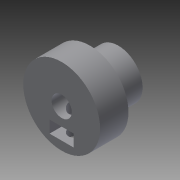
# Autodesk Inventor part: штука от моторчика2015
Saved by Autodesk Inventor 2015 (Build 190159000, 159)
## iProperties
Created: 2016-04-10
Part Number: штука от моторчика2015
Material: Generic
Document SubType Name: Modeling
Designer: 1
Density: 1 g/cm^3
Appearance: Default
Author: 1
Autodesk Inventor part; units mm, degrees
ref_plane "YZ Plane" through (0, 0, 0) normal (1, 0, 0) x (0, 1, 0)
ref_plane "XZ Plane" through (0, 0, 0) normal (0, 1, 0) x (-1, 0, 0)
ref_plane "XY Plane" through (0, 0, 0) normal (0, 0, 1) x (1, 0, 0)
sketch "Sketch1" plane through (0, 0, 0) normal (0, 1, 0) x (-1, 0, 0)
  circle A0 centre (0, 0) radius 6
  dimension "d0" = 12
  constraints: 1 centre point, 1 coincident
  measures "d0" diameter of A0
extrude "Extrusion1" add sketch "Sketch1" along normal blind 4 and the other way blind 3
sketch "Sketch2" plane through (0, -3, 0) normal (0, -1, 0) x (1, 0, 0)
  circle A0 centre (0, 0) radius 9.5
  dimension "d3" = 19
  constraints: 1 centre point, 1 coincident
  measures "d3" diameter of A0
extrude "Extrusion2" add sketch "Sketch2" along normal blind 7
sketch "Sketch7" plane through (0, 0, 0) normal (0, 0, 1) x (1, 0, 0)
  point P0 (0, 0)
sketch "Sketch9" plane through (0, 0, 0) normal (0, 0, 1) x (1, 0, 0)
  circle A0 centre (0, -6.5) radius 1.75
  line L0 (-9.5, -10) -> (9.5, -10) projected
  line L1 (0, -10) -> (0, -3)
  line L2 (0, -10) -> (0, -3)
  line L3 (-6, -3) -> (6, -3) projected
  point P0 (0, 0)
  dimension "d22" = 3.5
  constraints: 4 end point, 4 midpoint, 1 centre point, 1 coincident, 1 perpendicular
  measures "d22" diameter of A0
extrude "Extrusion8" cut sketch "Sketch9" against normal up to next
sketch "Sketch10" plane through (0, 4, 0) normal (0, 1, 0) x (1, 0, 0)
  circle A0 centre (0, 0) radius 2.5
  dimension "d26" = 5
  constraints: 1 centre point, 1 coincident
  measures "d26" diameter of A0
extrude "Extrusion9" cut sketch "Sketch10" against normal through all
sketch "Sketch11" plane through (0, -10, 0) normal (0, -1, 0) x (1, 0, 0)
  line L0 (3, -7.3359) -> (-3, -7.3359)
  line L1 (-3, -7.3359) -> (-3, -4.3359)
  line L2 (-3, -4.3359) -> (3, -4.3359)
  line L3 (3, -4.3359) -> (3, -7.3359)
  circle A0 centre (0, 0) radius 9.5 projected
  circle A1 centre (0, 0) radius 2.5 projected
  line L4 (0, -2.5) -> (0, -9.5)
  line L5 (4.4339, -2.3359) -> (-4.4946, -2.3359)
  line L6 (-4.4946, -2.3359) -> (-4.4946, -9.3359)
  line L7 (-4.4946, -9.3359) -> (4.4339, -9.3359)
  line L8 (4.4339, -9.3359) -> (4.4339, -2.3359)
  line L9 (-3, -5.8359) -> (3, -5.8359)
  dimension "d29" = 6
  dimension "d30" = 3
  dimension "d34" = 3.5
  constraints: 20 end point, 4 parallel, 2 horizontal, 2 midpoint, 2 perpendicular, 2 vertical alignment, 1 vertical, 2 other
  measures "d29" distance of L1.end L2.end
  measures "d30" distance of L0.end L1.end
  measures "d34" distance between parallel lines of L9 L5
extrude "Extrusion10" cut sketch "Sketch11" against normal blind 7 contours L0 L4 L9 L3 | L0 L1 L9 L4 | L9 L4 L2 L3 | L9 L1 L2 L4
body "Solid1"
